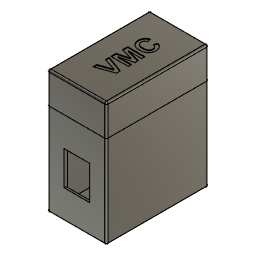
box-vmc v20 (Autodesk Fusion 360 design; units mm, degrees)
Autodesk Fusion 360 part; units mm, degrees
sketch "Sketch1" plane through (0, 0, 0) normal (0, 0, 1) x (1, 0, 0)
  line L0 (17, 29.5) -> (-17, 29.5)
  line L1 (-17, 29.5) -> (-17, -29.5)
  line L2 (-17, -29.5) -> (17, -29.5)
  line L3 (17, -29.5) -> (17, 29.5)
  line L4 (17, 29.5) -> (-17, -29.5) construction
  line L5 (-17, 29.5) -> (17, -29.5) construction
  dimension "d6" = 34
  dimension "d7" = 59
  constraint horizontal L0
  constraint perpendicular L0 L1
  constraint parallel L0 L2
  constraint parallel L1 L3
  constraint coincident L4 origin
  constraint coincident L5 origin
  measures "d6" distance of L1.end L2.end
  measures "d7" distance of L0.end L1.end
extrude "Extrude1" add sketch "Sketch1" along normal blind 71.4 contours L0 L1 L2 L3 picked at (-5.666667, -9.833333) makes body 1
shell "Shell1" thickness 2 removed faces 0 bodies 1
sketch "Sketch2" plane through (-15, 0, 0) normal (1, 0, 0) x (0, 1, 0)
  line L0 (-27.5, 2) -> (27.5, 2)
  line L1 (27.5, 2) -> (27.5, 69.4)
  line L2 (27.5, 69.4) -> (-27.5, 69.4)
  line L3 (-27.5, 69.4) -> (-27.5, 2)
  line L4 (3.971831, 69.4) -> (5.6, 69.4)
  line L5 (5.6, 69.4) -> (5.6, 2)
  line L6 (5.6, 2) -> (3.971831, 2)
  line L7 (3.971831, 2) -> (3.971831, 69.4)
  dimension "d11" = 21.9
  constraint horizontal L4
  constraint vertical L5
  constraint horizontal L6
  constraint vertical L7
  constraint coincident L0 L5.end
  measures "d11" distance of L1.end L4.end
extrude "Extrude2" add sketch "Sketch2" along normal blind 3 contours L0 L2 L4 L5 L6 L7 picked at (4.514554, 46.933333) bodies 1
sketch "Sketch3" plane through (0, 5.6, 0) normal (0, 1, 0) x (-1, 0, 0)
  line L0 (15, 2) -> (15, 69.4)
  line L1 (15, 69.4) -> (12, 69.4)
  line L2 (12, 69.4) -> (12, 2)
  line L3 (12, 2) -> (15, 2)
  point P0 (12, 35.7)
  point P1 (15, 35.7)
  point P2 (13.5, 69.4)
  point P3 (13.5, 2)
  constraint midpoint L2 P0
  constraint midpoint L0 P1
  constraint midpoint L1 P2
  constraint midpoint L3 P3
sketch "Sketch4" plane through (0, 5.6, 0) normal (0, 1, 0) x (-1, 0, 0)
  line L0 (13.000006, 37.822633) -> (13.000006, 1.994904)
  line L1 (13.000006, 37.822633) -> (11.973423, 37.822633)
  line L2 (11.973423, 37.822633) -> (11.973423, 1.994904)
  line L3 (11.973423, 1.994904) -> (13.000006, 1.994904)
  point P0 (15, 2)
  point P1 (15, 69.4)
  point P2 (12, 69.4)
  dimension "d74" = 2
  constraint perpendicular L0 L1
  constraint perpendicular L1 L2
  constraint perpendicular L0 L3
  constraint vertical L2
sketch "Sketch6" plane through (0, 27.5, 0) normal (0, -1, 0) x (1, 0, 0)
  line L0 (-15, 2) -> (15, 2)
  line L1 (-15, 69.4) -> (-15, 2)
  line L2 (-13.000006, 37.822633) -> (-13.000006, 1.994904)
  line L3 (-11.973423, 37.822633) -> (-11.973423, 1.994904)
  line L4 (-13.000006, 37.822633) -> (-11.973423, 37.822633)
  line L5 (-11.973423, 1.994904) -> (-13.000006, 1.994904)
extrude "Extrude4" add sketch "Sketch4" along normal blind 1 contours L0 L1 L2 L3 picked at (12.315618, 13.93748) bodies 1
sketch "Sketch7" plane through (0, 0, 2) normal (0, 0, 1) x (-1, 0, 0)
  line L0 (-15, -27.5) -> (15, -27.5)
  line L1 (15, -3.971831) -> (15, 27.5)
  line L2 (15, -5.6) -> (13.000006, -5.6)
  line L3 (13.000006, -5.6) -> (13.000006, -6.6)
  line L4 (11.973423, -6.6) -> (11.973423, -5.6)
  line L5 (12, -3.971831) -> (15, -3.971831)
  line L6 (15, 27.5) -> (-15, 27.5)
  line L7 (-15, 27.5) -> (-15, -27.5)
  line L8 (1.005715, -4.371831) -> (1.005715, 27.5) construction
  line L9 (13.000006, -6.6) -> (11.973423, -6.6)
  line L10 (11.973423, -5.6) -> (12, -5.6)
  line L11 (12, -5.6) -> (12, -3.971831)
  line L12 (15, -27.5) -> (15, -5.6)
  dimension "d26" = 14
  constraint perpendicular L6 L8
sketch "Sketch10" plane through (0, 0, 2) normal (0, 0, 1) x (-1, 0, 0)
  line L0 (-7.4, -25.5) -> (-9.4, -25.5)
  line L1 (-9.4, -25.5) -> (-9.4, 5.5)
  line L2 (-9.4, 5.5) -> (-7.4, 5.5)
  line L3 (-7.4, 5.5) -> (-7.4, -25.5)
  point P0 (-15, -27.5)
  dimension "d37" = 2
  dimension "d38" = 31
  dimension "d39" = 2
  dimension "d40" = 5.6
  constraint horizontal L0
  constraint vertical L1
  constraint horizontal L2
  constraint vertical L3
  measures "d37" distance of L0.start L0.end
  measures "d38" distance of L0.start L2.end
  measures "d39" vertical distance of L0.end P0
  measures "d40" horizontal distance of L0.end P0
extrude "Extrude8" add sketch "Sketch10" along normal blind 7 contours L0 L1 L2 L3 picked at (-8.066667, -4.833333) bodies 1
fillet "Fillet2" radius 1 1 faces at (8.066667, 4.833333, 9) on bodies 1
fillet "Fillet3" radius 2 1 edges at (7.4, 10, 2) on bodies 1
ref_plane "WorkPlane1" through (0, 0, 51.4) normal (0, 0, 1) x (1, 0, 0)
fillet "Fillet4" radius 1 12 edges at (17, -29.5, 35.7) (-17, -29.5, 35.7) (0, -29.5, 0) (17, 0, 0) (-17, 0, 0) (0, 29.5, 0) (17, 29.5, 35.7) (-17, 29.5, 35.7) (0, -29.5, 71.4) (-17, 0, 71.4) (0, 29.5, 71.4) (17, 0, 71.4) on bodies 1
split "Split1" by plane through (0, 0, 51.4) normal (0, 0, 1) bodies 1 makes body 2 at (-5.333333, -9.5, 71.4)
sketch "Sketch11" plane through (0, 0, 51.4) normal (0, 0, 1) x (-1, 0, 0)
  arc A0 (16, -29.5) -> (17, -28.5) centre (16, -28.5) ccw
  line L0 (17, -28.5) -> (17, 28.5)
  arc A1 (17, 28.5) -> (16, 29.5) centre (16, 28.5) ccw
  line L1 (16, 29.5) -> (-16, 29.5)
  arc A2 (-16, 29.5) -> (-17, 28.5) centre (-16, 28.5) ccw
  line L2 (-17, 28.5) -> (-17, -28.5)
  arc A3 (-17, -28.5) -> (-16, -29.5) centre (-16, -28.5) ccw
  line L3 (-16, -29.5) -> (16, -29.5)
  line L4 (15, -3.971831) -> (12, -3.971831)
  line L5 (12, -3.971831) -> (12, -5.6)
  line L6 (12, -5.6) -> (15, -5.6)
  line L7 (15, -5.6) -> (15, -27.5)
  line L8 (15, -27.5) -> (-15, -27.5)
  line L9 (-15, -27.5) -> (-15, 27.5)
  line L10 (-15, 27.5) -> (15, 27.5)
  line L11 (15, 27.5) -> (15, -3.971831)
  line L12 (16, 28.5) -> (-16, 28.5)
  line L13 (-16, 28.5) -> (-16, -28.5)
  line L14 (-16, -28.5) -> (16, -28.5)
  line L15 (16, -28.5) -> (16, 28.5)
  line L16 (15, 27.5) -> (-15, 27.5)
  line L17 (-15, 27.5) -> (-15, -27.5)
  line L18 (-15, -27.5) -> (15, -27.5)
  line L19 (15, -27.5) -> (15, 27.5)
  line L20 (16, 28.7) -> (-16, 28.7)
  arc A4 (-16, 28.7) -> (-16.2, 28.5) centre (-16, 28.5) ccw
  line L21 (-16.2, 28.5) -> (-16.2, -28.5)
  arc A5 (-16.2, -28.5) -> (-16, -28.7) centre (-16, -28.5) ccw
  line L22 (-16, -28.7) -> (16, -28.7)
  arc A6 (16, -28.7) -> (16.2, -28.5) centre (16, -28.5) ccw
  line L23 (16.2, -28.5) -> (16.2, 28.5)
  arc A7 (16.2, 28.5) -> (16, 28.7) centre (16, 28.5) ccw
  dimension "d50" = -1
  dimension "d52" = -0.8
extrude "Extrude9" add sketch "Sketch11" along normal blind 2 contours A0 L0 A1 L1 A2 L2 A3 L3 picked at (-16.733333, -9.5) bodies 1
sketch "Sketch12" plane through (0, 0, 51.4) normal (0, 0, -1) x (1, 0, 0)
  line L0 (-12, -3.971831) -> (-15, -3.971831)
  line L1 (-15, -3.971831) -> (-15, 27.5)
  line L2 (-15, 27.5) -> (15, 27.5)
  line L3 (15, 27.5) -> (15, -27.5)
  line L4 (15, -27.5) -> (-15, -27.5)
  line L5 (-15, -27.5) -> (-15, -5.6)
  line L6 (-15, -5.6) -> (-12, -5.6)
  line L7 (-12, -5.6) -> (-12, -3.971831)
  arc A0 (-17, -28.5) -> (-16, -29.5) centre (-16, -28.5) ccw
  line L8 (-16, -29.5) -> (16, -29.5)
  arc A1 (16, -29.5) -> (17, -28.5) centre (16, -28.5) ccw
  line L9 (17, -28.5) -> (17, 28.5)
  arc A2 (17, 28.5) -> (16, 29.5) centre (16, 28.5) ccw
  line L10 (16, 29.5) -> (-16, 29.5)
  arc A3 (-16, 29.5) -> (-17, 28.5) centre (-16, 28.5) ccw
  line L11 (-17, 28.5) -> (-17, -28.5)
  line L12 (-15, -27.5) -> (-15, 27.5)
  line L13 (-16, -28.5) -> (-16, 28.5)
  line L14 (16, -28.5) -> (-16, -28.5)
  line L15 (15, -27.5) -> (-15, -27.5)
  line L16 (16, 28.5) -> (16, -28.5)
  line L17 (15, 27.5) -> (15, -27.5)
  line L18 (-15, 27.5) -> (15, 27.5)
  line L19 (-16, 28.5) -> (16, 28.5)
extrude "Extrude11" cut sketch "Sketch12" against normal blind 2 contours A0 L8 A1 L9 A2 L10 A3 L11 picked at (-16.333333, -9.5) bodies 2
sketch "Sketch13" plane through (0, 0, 71.4) normal (0, 0, 1) x (-1, 0, 0)
  line L0 (-16, 28.5) -> (-16, -28.5)
  line L1 (-16, -28.5) -> (16, -28.5)
  line L2 (16, -28.5) -> (16, 28.5)
  line L3 (16, 28.5) -> (-16, 28.5)
  line L4 (-7, 20.5) -> (-7, -20.5) construction
  line L5 (-7, -20.5) -> (7, -20.5) construction
  line L6 (7, -20.5) -> (7, 20.5) construction
  line L7 (7, 20.5) -> (-7, 20.5) construction
  dimension "d59" = 8
  dimension "d60" = 8
  dimension "d61" = 9
  dimension "d62" = 9
  dimension "d63" = 9
  dimension "d64" = 9
  text T0 "VMC" font "Arial" height 10 bold align centre middle in box 41 x 14 at (-7, 20.5) x (0, -1) y (1, 0) spacing 1 kerned
  measures "d59" distance of L2.end
  measures "d60" distance of L1.end
  measures "d61" distance of L2.end
  measures "d62" distance of L0.start
  measures "d63" distance of L0.end
  measures "d64" distance of L1.end
extrude "Extrude12" cut sketch "Sketch13" against normal blind 0.4 text T0 bodies 2
sketch "Sketch14" plane through (0, -27.5, 0) normal (0, 1, 0) x (-1, 0, 0)
  line L0 (15, 51.4) -> (-15, 51.4)
  line L1 (-15, 51.4) -> (-15, 2)
  line L2 (-15, 2) -> (15, 2)
  line L3 (15, 2) -> (15, 51.4)
  line L4 (15, 2) -> (-15, 51.4) construction
  line L5 (15, 51.4) -> (-15, 2) construction
  line L6 (7.4, 36.5) -> (-7.4, 36.5)
  line L7 (-7.4, 36.5) -> (-7.4, 16.9)
  line L8 (-7.4, 16.9) -> (7.4, 16.9)
  line L9 (7.4, 16.9) -> (7.4, 36.5)
  line L10 (7.4, 36.5) -> (-7.4, 16.9) construction
  line L11 (-7.4, 36.5) -> (7.4, 16.9) construction
  point P0 (0, 26.7)
  dimension "d67" = 14.8
  dimension "d68" = 19.6
  constraint coincident L2.end L3.start
  constraint coincident L0.end L1.start
  constraint coincident L0.start L3.end
  constraint coincident L1.end L2.start
  constraint horizontal L6
  constraint perpendicular L6 L7
  constraint parallel L6 L8
  constraint parallel L7 L9
  constraint coincident L10 P0
  constraint coincident L11 P0
  constraint midpoint L4 P0
  measures "d67" distance of L7.end L8.end
  measures "d68" distance of L6.end L7.end
extrude "Extrude13" cut sketch "Sketch14" against normal through all contours L6 L7 L8 L9 picked at (-2.466667, 29.966667) bodies 1
chamfer "Chamfer2" distance 0.8 angle 45 1 edges at (0, -27.5, 16.9) on bodies 1
extrude "Extrude14" add sketch "Sketch6" along normal blind 1 contours L0 L2 L3 L4 picked at (-12.315618, 13.940878) bodies 1
sketch "Sketch15" plane through (15, 0, 0) normal (-1, 0, 0) x (0, -1, 0)
  line L0 (27.5, 51.4) -> (-27.5, 51.4)
  line L1 (-27.5, 51.4) -> (-27.5, 2)
  line L2 (-27.5, 2) -> (27.5, 2)
  line L3 (27.5, 2) -> (27.5, 51.4)
  line L4 (6.1, 2) -> (8.1, 2)
  line L5 (8.1, 2) -> (8.1, 38.4)
  line L6 (8.1, 38.4) -> (6.1, 38.4)
  line L7 (6.1, 38.4) -> (6.1, 2)
  dimension "d80" = 2
  dimension "d81" = 33.6
  constraint horizontal L4
  constraint vertical L5
  constraint horizontal L6
  constraint vertical L7
  constraint coincident L2 L4.start
  measures "d80" distance of L4.start L4.end
  measures "d81" distance of L1.end L4.start
extrude "Extrude15" add sketch "Sketch15" along normal blind 6 separate body contours L2 L4 L5 L6 L7 picked at (6.766667, 26.266667) makes body 3
combine "Combine2" operation add target body 1 tool bodies 3
sketch "Sketch16" plane through (0, -6.1, 0) normal (0, 1, 0) x (-1, 0, 0)
  line L0 (-15, 38.4) -> (-15, 2)
  line L1 (-15, 2) -> (-9.4, 2)
  line L2 (-9, 8.8) -> (-9, 38.4)
  line L3 (-9, 38.4) -> (-15, 38.4)
  line L4 (-9, 38.4) -> (-11.6, 38.400009)
  line L5 (-11.6, 38.400009) -> (-11.6, 2.000276)
  line L6 (-11.6, 2.000276) -> (-9, 2.000232)
  line L7 (-9, 2.000232) -> (-9, 38.4)
  line L8 (-9.4, 2) -> (-9.4, 8)
  arc A0 (-9, 8.8) -> (-9.4, 8) centre (-8.4, 8) ccw
  line L9 (-9, 2) -> (-9, 38.4)
  line L10 (-9, 38.4) -> (-15, 38.4)
  line L11 (-15, 38.4) -> (-15, 2)
  line L12 (-15, 2) -> (-9, 2)
  dimension "d85" = 3.4
  dimension "d86" = 3.4
  constraint vertical L7
  constraint coincident L2.end L3.start
extrude "Extrude16" add sketch "Sketch16" along normal blind 1 contours L2 L3 L4 L5 L6 L7 L8 A0 L9 L10 | L6 L7 L8 A0 L9 picked at (-9.866667, 28.533333) picked at (-9.133333, 6.266744) bodies 1
fillet "Fillet6" radius 0.5 1 edges at (11.6, -5.1, 20.200138) on bodies 1
fillet "Fillet6" radius 1 1 edges at (9, -8.1, 20.2) on bodies 1
sketch "Sketch17" plane through (-16.2, 0, 0) normal (1, 0, 0) x (0, 1, 0)
  line L0 (-28.5, 51.4) -> (28.5, 51.4)
  line L1 (28.5, 51.4) -> (28.5, 53.4)
  line L2 (28.5, 53.4) -> (-28.5, 53.4)
  line L3 (-28.5, 53.4) -> (-28.5, 51.4)
sketch "Sketch19" plane through (-16.2, 0, 0) normal (1, 0, 0) x (0, 1, 0)
  circle A0 centre (4.5, 52.4) radius 0.7
  line L0 (28.5, 53.4) -> (-28.5, 53.4)
  line L1 (-28.5, 51.4) -> (28.5, 51.4)
  dimension "d93" = 1.4
  dimension "d94" = 1
  dimension "d95" = 1
  measures "d93" diameter of A0
  measures "d94" distance of A0.centre L0
  measures "d95" distance of A0.centre L1
sketch "Sketch20" plane through (16.2, 0, 0) normal (-1, 0, 0) x (0, -1, 0)
  line L0 (-28.5, 51.4) -> (28.5, 51.4)
  line L1 (28.5, 51.4) -> (28.5, 53.4)
  line L2 (28.5, 53.4) -> (-28.5, 53.4)
  line L3 (-28.5, 53.4) -> (-28.5, 51.4)
  circle A0 centre (-4.5, 52.4) radius 0.7
  point P0 (-4.5, 52.4)
extrude "Extrude17" add sketch "Sketch20" along normal blind 0.4 contours A0 picked at (-4.551922, 52.627483) bodies 1
extrude "Extrude18" add sketch "Sketch19" along normal blind 0.4 contours A0 picked at (4.448079, 52.627483) bodies 1
fillet "Fillet7" radius 0.4 1 edges at (15.8, 5.152629, 52.146869) on bodies 1
fillet "Fillet8" radius 0.4 1 edges at (-15.8, 3.847371, 52.146869) on bodies 1
combine "Combine3" operation cut target body 2 tool bodies 1 keep tools
extrude "Extrude19" cut sketch "Sketch19" along normal blind 0.5 contours A0 picked at (4.448079, 52.627483) bodies 2
extrude "Extrude20" cut sketch "Sketch20" along normal blind 0.5 contours A0 picked at (-4.551922, 52.627483) bodies 2
chamfer "Chamfer3" distance 0.1 angle 45 2 edges at (16, 5.152629, 52.146869) (-16, 3.847371, 52.146869) on bodies 2
equation "innerLength = 30 mm"
equation "innerWidth = 55 mm"
equation "innerHeight = 67 mm + tollerance * 2"
equation "tollerance = 0.2 mm"
equation "shell = 2 mm"
equation "d6 = innerLength + shell * 2"
equation "d7 = innerWidth + shell * 2"
equation "d8 = innerHeight + shell * 2"
equation "d10 = shell"
equation "d11 = 21.5 mm + tollerance * 2"
equation "d51 = -shell"
equation "d52 = -1 mm + tollerance"
